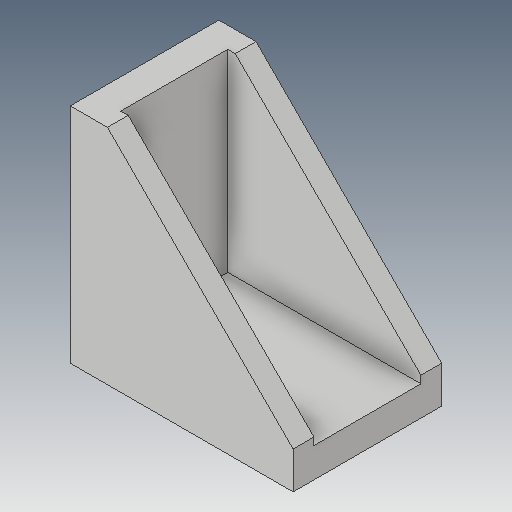
# Autodesk Inventor part: ブラケット2
Saved by Autodesk Inventor 2020.3 (Build 243373000, 373)
## iProperties
Part Number: ブラケット2
Material: 一般
Document SubType Name: Modeling
Designer: highs
Density: 1 g/cm^3
Appearance: 既定
Description: https://jp.misumi-ec.com/vona2/detail/110300437260/?HissuCode=HBLFSN5-SEP&PNSearch=HBLFSN5-SEP&KWSearch=HBLFSN5-SEP&searchFlow=results2products
Stock Number: 数はナビトンに準魚
Author: highs
Revision Number: 4個では絶対足らない．
Autodesk Inventor part; units mm, degrees
ref_plane "YZ Plane" through (0, 0, 0) normal (1, 0, 0) x (0, 1, 0)
ref_plane "XZ Plane" through (0, 0, 0) normal (0, 1, 0) x (-1, 0, 0)
ref_plane "XY Plane" through (0, 0, 0) normal (0, 0, 1) x (1, 0, 0)
sketch "スケッチ1" plane through (0, 0, 0) normal (0, 0, 1) x (1, 0, 0)
  line L0 (0, 0) -> (30, 0)
  line L1 (30, 0) -> (30, 5)
  line L2 (30, 5) -> (5, 30)
  line L3 (5, 30) -> (0, 30)
  line L4 (0, 30) -> (0, 0)
  dimension "d0" = 30
  dimension "d1" = 30
  dimension "d2" = 5
  constraints: 10 end point, 3 perpendicular, 1 horizontal, 1 parallel
  measures "d0" distance of L0.start L0.end
  measures "d1" distance of L3.end L0.start
  measures "d2" distance of L0.end L1.end
extrude "押し出し1" add sketch "スケッチ1" along normal blind 20
sketch "スケッチ2" plane through (30, 0, 0) normal (1, 0, 0) x (0, 0, -1)
  line L0 (0, 30) -> (-20, 30) projected
  line L1 (-17.2, 30) -> (-2.8, 30)
  line L2 (-2.8, 30) -> (-2.8, 4)
  line L3 (-2.8, 4) -> (-17.2, 4)
  line L4 (-17.2, 4) -> (-17.2, 30)
  line L5 (0, 0) -> (-20, 0) projected
  line L6 (0, 30) -> (0, 0) projected
  line L7 (-20, 5) -> (-20, 30) projected
  dimension "d5" = 4
  dimension "d6" = 2.8
  dimension "d7" = 2.8
  constraints: 8 end point, 2 parallel, 1 horizontal, 1 perpendicular, 1 point on line
  measures "d5" distance between parallel lines of L5 L3
  measures "d6" distance between parallel lines of L6 L2
  measures "d7" distance between parallel lines of L7 L4
extrude "押し出し2" cut sketch "スケッチ2" against normal blind 26
